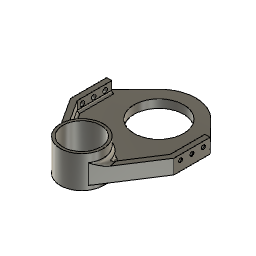
JRCNC0011 v29 (Autodesk Fusion 360 design; units mm, degrees)
Autodesk Fusion 360 part; units mm, degrees
sketch "Sketch1" plane through (0, 0, 0) normal (0, 0, 1) x (1, 0, 0)
  line L0 (0, -20.75) -> (0, 110.05) construction
  line L1 (-20.3398, -4.1055) -> (-34.7982, 67.5262)
  arc A0 (34.7982, 67.5262) -> (-34.7982, 67.5262) centre (0, 74.55) ccw
  line L2 (20.3398, -4.1055) -> (34.7982, 67.5262)
  arc A1 (-20.3398, -4.1055) -> (20.3398, -4.1055) centre (0, 0) ccw
  circle A2 centre (0, 74.55) radius 35.5
  circle A3 centre (0, 0) radius 20.75
  circle A4 centre (0, 74.55) radius 24
  circle A5 centre (0, 0) radius 18.25
  line L3 (-20.6187, 2.3305) -> (-32.1626, 59.5228)
  line L4 (20.6187, 2.3305) -> (32.1626, 59.5228)
  dimension "d4" = 130.8
  dimension "d15" = 71
  dimension "d16" = 41.5
  dimension "d17" = 48
  dimension "d18" = 36.5
  dimension "d65" = 1
  constraint vertical L0
  constraint coincident A1.centre L0
  constraint tangent L2 A1
  constraint tangent A0 L2
  constraint tangent L1 A0
  constraint tangent L1 A1
  constraint concentric A0 A2
  constraint coincident L0.end A2
  constraint coincident A1.centre A3.centre
  constraint coincident L0.start A3
  constraint coincident L0 A0.centre
  constraint coincident L1.end A2
  constraint coincident L1.start A3
  constraint concentric A2 A4
  constraint concentric A3 A5
  constraint coincident A3 L3.start
  constraint coincident A2 L3.end
  constraint symmetric L0 L3.start L4.start
  constraint symmetric L0 L3.end L4.end
  constraint parallel L1 L3
  measures "d4" distance of L0.start L0.end
  measures "d15" diameter of A2
  measures "d16" diameter of A3
  measures "d17" diameter of A4
  measures "d18" diameter of A5
  measures "d65" distance of L1 L3
extrude "Extrude1" add sketch "Sketch1" along normal blind 4 contours A1 A3 | A0 A2 | A2 A3 L3 L4
sketch "Sketch3" plane through (0, 0, 4) normal (0, 0, 1) x (-1, 0, 0)
  circle A0 centre (0, -74.55) radius 24
  circle A1 centre (0, 0) radius 18.25
  arc A2 (-32.1626, -59.5228) -> (32.1626, -59.5228) centre (0, -74.55) ccw
  arc A3 (20.6187, -2.3305) -> (-20.6187, -2.3305) centre (0, 0) ccw
  circle A4 centre (0, 0) radius 20.75
  circle A5 centre (0, 0) radius 18.25
  line L0 (-20.6187, -2.3305) -> (-32.1626, -59.5228)
  line L1 (32.1626, -59.5228) -> (20.6187, -2.3305)
  constraint coincident A1.centre A3.centre
  constraint equal A3 A4
  constraint equal A1 A5
extrude "Extrude4" add sketch "Sketch3" along normal blind 27 contours A3 A4
sketch "Sketch2" plane through (0, 0, 4) normal (0, 0, 1) x (-1, 0, 0)
  line L0 (-50, -110.05) -> (50, -110.05)
  line L1 (50, -110.05) -> (50, -39.05)
  line L2 (50, -39.05) -> (-50, -39.05)
  line L3 (-50, -39.05) -> (-50, -110.05)
  line L4 (-50, -110.05) -> (50, -39.05) construction
  line L5 (50, -110.05) -> (-50, -39.05) construction
  arc A0 (-20.6187, -2.3305) -> (20.6187, -2.3305) centre (0, 0) ccw
  arc A1 (-32.1626, -59.5228) -> (32.1626, -59.5228) centre (0, -74.55) ccw
  circle A2 centre (0, -74.55) radius 24
  line L6 (25.4525, -99.2972) -> (50, -74.05)
  circle A3 centre (0, 0) radius 20.75
  line L7 (17.4183, 11.2767) -> (50, -39.05)
  line L8 (0, -110.05) -> (0, 0) construction
  line L9 (-17.4183, 11.2767) -> (-50, -39.05)
  line L10 (-25.4525, -99.2972) -> (-50, -74.05)
  line L11 (0, -74.55) -> (50.0155, -74.55) construction
  line L12 (-20.6187, -2.3305) -> (-32.1626, -59.5228)
  line L13 (32.1626, -59.5228) -> (20.6187, -2.3305)
  point P0 (0, -74.55)
  point P1 (0, -110.05)
  dimension "d21" = 100
  dimension "d32" = 35
  constraint horizontal L0
  constraint perpendicular L0 L1
  constraint parallel L0 L2
  constraint parallel L1 L3
  constraint coincident L4 P0
  constraint coincident L5 P0
  constraint midpoint L0 P1
  constraint midpoint P1 A1
  constraint coincident P0 A1.centre
  constraint coincident A1 L6.start
  constraint coincident L1 L6.end
  constraint tangent A1 L6
  constraint coincident A3 L7.start
  constraint coincident L1 L2.start
  constraint tangent A3 L7
  constraint coincident P1 L8.start
  constraint coincident A0.centre A3.centre
  constraint symmetric L6.start L8 L10.start
  constraint symmetric L6.end L8 L10.end
  constraint symmetric L7.start L8 L9.start
  constraint symmetric L1.end L8 L2.end
  constraint perpendicular L1 L11
  constraint coincident L1.end L2.start
  measures "d21" distance of L0.start L0.end
  measures "d32" distance of L6.end L1.end
extrude "Extrude3" add sketch "Sketch2" along normal blind 4 contours L2 A1 L12 L13 | L2 L3 A1 L10 L12 | L1 L2 A1 L6 L13 | L2 A3 L9 L12 | L2 A0 A3 L12 L13 | L2 A3 L7 L13
sketch "Sketch4" plane through (0, 0, 8) normal (0, 0, 1) x (-1, 0, 0)
  line L0 (-50, -39.05) -> (-50, -74.05)
  line L1 (50, -74.05) -> (50, -39.05)
  circle A0 centre (0, -74.55) radius 26
  line L2 (-50, -74.05) -> (-45, -74.05)
  line L3 (-45, -74.05) -> (-45, -39.05)
  line L4 (-45, -39.05) -> (-50, -39.05)
  line L5 (-50, -39.05) -> (-50, -74.05)
  line L6 (50, -74.05) -> (45, -74.05)
  line L7 (45, -74.05) -> (45, -39.05)
  line L8 (45, -39.05) -> (50, -39.05)
  line L9 (50, -39.05) -> (50, -74.05)
  line L10 (-50, -74.05) -> (-25.4525, -99.2972)
  arc A1 (-25.4525, -99.2972) -> (25.4525, -99.2972) centre (0, -74.55) ccw
  line L11 (25.4525, -99.2972) -> (50, -74.05)
  arc A2 (-17.4183, 11.2767) -> (17.4183, 11.2767) centre (0, 0) ccw
  line L12 (45, -74.05) -> (45, -79.1925)
  line L13 (45, -79.1925) -> (50, -74.05)
  line L14 (-45, -74.05) -> (-45, -79.1925)
  line L15 (-45, -79.1925) -> (-50, -74.05)
  arc A3 (-22.1428, -5.2212) -> (22.1428, -5.2212) centre (0, 0) ccw
  line L16 (45, -40.5272) -> (22.1428, -5.2212)
  line L17 (45, -72.02) -> (45, -40.5272)
  line L18 (21.8676, -95.8116) -> (45, -72.02)
  arc A4 (-21.8676, -95.8116) -> (21.8676, -95.8116) centre (0, -74.55) ccw
  line L19 (-45, -72.02) -> (-21.8676, -95.8116)
  line L20 (-45, -40.5272) -> (-45, -72.02)
  line L21 (-22.1428, -5.2212) -> (-45, -40.5272)
  line L22 (-17.4183, 11.2767) -> (-50, -39.05)
  line L23 (50, -39.05) -> (17.4183, 11.2767)
  circle A5 centre (0, -74.55) radius 24
  line L24 (25.4525, -99.2972) -> (50, -74.05)
  line L25 (50, -74.05) -> (50, -39.05)
  line L26 (50, -39.05) -> (17.4183, 11.2767)
  arc A6 (-17.4183, 11.2767) -> (17.4183, 11.2767) centre (0, 0) ccw
  line L27 (-17.4183, 11.2767) -> (-50, -39.05)
  line L28 (-50, -39.05) -> (-50, -74.05)
  line L29 (-50, -74.05) -> (-25.4525, -99.2972)
  arc A7 (-25.4525, -99.2972) -> (25.4525, -99.2972) centre (0, -74.55) ccw
  dimension "d27" = 5
  dimension "d28" = 5
  dimension "d60" = 5
  dimension "d61" = 2
  dimension "d62" = 5
  dimension "d63" = 5
  dimension "d66" = 5
  dimension "d67" = 5
  constraint horizontal L2
  constraint vertical L3
  constraint horizontal L4
  constraint vertical L5
  constraint coincident L0.end L2.start
  constraint horizontal L6
  constraint vertical L7
  constraint horizontal L8
  constraint vertical L9
  constraint coincident L1.start L6.start
  constraint coincident L11 L12.end
  constraint perpendicular L6 L12
  constraint coincident L10 L14.end
  constraint perpendicular L2 L14
  constraint concentric A2 A3
  constraint parallel L1 L17
  constraint parallel L11 L18
  constraint parallel L10 L19
  constraint parallel L0 L20
  constraint tangent A4 L19
  constraint tangent L18 A4
  constraint coincident L0.start L4.end
  constraint coincident L1.end L8.end
  constraint parallel L16 L23
  constraint parallel L21 L22
  constraint coincident L7 L17.start
  constraint coincident L3 L19.start
  constraint concentric A0 A4
  measures "d27" distance of L1.start L6.end
  measures "d28" distance of L0.end L2.end
  measures "d60" distance of L11 L18
  measures "d61" distance of A2 A3
  measures "d62" distance of L16 L23
  measures "d63" distance of L21 L22
  measures "d66" distance of L10 L19
  measures "d67" distance of A1 A4
extrude "Extrude5" add sketch "Sketch4" along normal blind 10 contours L0 L2 L3 L4 L5 L20 L28 | L3 L4 L7 L8 A2 A3 L16 L21 L22 L23 L26 A6 L27 | L1 L6 L7 L8 L9 L17 L25
sketch "Sketch5" plane through (50, 0, 0) normal (1, 0, 0) x (0, 1, 0)
  line L0 (74.05, 18) -> (39.05, 18)
  line L1 (74.05, 13) -> (39.05, 13)
  line L2 (39.05, 18) -> (39.05, 4)
  line L3 (74.05, 8) -> (74.05, 18)
  line L4 (39.05, 4) -> (74.05, 4)
  line L5 (74.05, 4) -> (74.05, 8)
  point P0 (45.55, 13)
  point P1 (67.55, 13)
  point P2 (56.55, 13)
  dimension "d36" = 11
  dimension "d37" = 11
  dimension "d41" = 5
  constraint coincident L1 P0
  constraint coincident L1 P1
  constraint midpoint L1 P2
  measures "d36" distance of P0 P2
  measures "d37" distance of P1 P2
  measures "d41" distance of L0 L1
hole "Hole1" at (50, 45.55, 13) at (50, 56.55, 13) at (50, 67.55, 13) direction (-1, 0, 0) diameter 3.9 depth 101 tip angle 118
sketch "Sketch6" plane through (0, 0, 0) normal (0, 0, -1) x (-1, 0, 0)
  line L0 (20, 22.25) -> (-20, 22.25) construction
  line L1 (22, 32.25) -> (-22, 32.25) construction
  circle A0 centre (0, 0) radius 18.25
  circle A1 centre (0, 74.55) radius 24
  arc A2 (-20.6187, 2.3305) -> (20.6187, 2.3305) centre (0, 0) ccw
  arc A3 (32.1626, 59.5228) -> (-32.1626, 59.5228) centre (0, 74.55) ccw
  line L2 (0, -20.75) -> (0, 74.55) construction
  line L3 (20.6187, 2.3305) -> (32.1626, 59.5228)
  line L4 (-32.1626, 59.5228) -> (-20.6187, 2.3305)
  point P0 (0, 22.25)
  point P1 (0, 32.25)
  point P2 (0, 20.75)
  point P3 (0, -20.75)
  dimension "d46" = 40
  dimension "d47" = 44
  dimension "d58" = 43
  dimension "d59" = 10
  constraint midpoint L0 P0
  constraint midpoint L1 P1
  constraint midpoint A2 P3
  constraint coincident P3 L2.start
  constraint vertical L2
  constraint coincident P0 L2
  constraint coincident P1 L2
  constraint horizontal L1
  constraint coincident A1.centre A3.centre
  measures "d46" distance of L0.start L0.end
  measures "d47" distance of L1.start L1.end
  measures "d58" distance of P0 P3
  measures "d59" distance of P0 P1
hole "Hole2" at (-22, 32.25, 0) at (22, 32.25, 0) at (20, 22.25, 0) at (-20, 22.25, 0) direction (0, 0, 1) diameter 8.5 depth 3.5 tip angle 180
sketch "Sketch7" plane through (50, 0, 0) normal (1, 0, 0) x (0, 1, 0)
  line L0 (50.55, 8) -> (98.55, 8)
  line L1 (74.55, 8) -> (74.55, 18)
  constraint midpoint L0 L1.start
  constraint perpendicular L0 L1
fillet "Fillet2" radius 5 1 edges at (0, 20.75, 18)
fillet "Fillet4" radius 2 5 edges at (-33.5714, 22.8742, 8) (0, 22.75, 8) (33.5714, 22.8742, 8) (45, 57.2886, 8) (-45, 57.2886, 8)
sketch "Sketch8" plane through (-45, 0, 0) normal (1, 0, 0) x (0, 1, 0)
  line L0 (40.5272, 10) -> (74.05, 10)
  line L1 (74.05, 10) -> (74.05, 18)
  line L2 (74.05, 18) -> (40.5272, 18)
  line L3 (40.5272, 18) -> (40.5272, 10)
  circle A0 centre (67.55, 13) radius 1.95
  circle A1 centre (45.55, 13) radius 1.95
  circle A2 centre (56.55, 13) radius 1.95
hole "Hole3" at (-45, 45.55, 13) at (-45, 56.55, 13) at (-45, 67.55, 13) direction (-1, 0, 0) diameter 4.496 depth 4 tip angle 180
mirror "Mirror1" about plane through (0, 0, 0) normal (1, 0, 0) of "Hole3"
equation "d41 = ( 10 / 2 ) * 1 mm"
